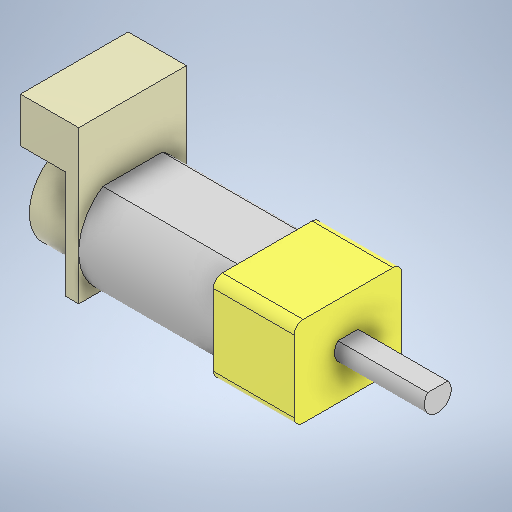
# Autodesk Inventor part: motor
Saved by Autodesk Inventor 2025.2 (Build 292293000, 293)
## iProperties
Created: 2025-06-11
Part Number: motor
Material: Generic
Document SubType Name: Modeling
Designer: cdavi
Density: 1 g/cm^3
Appearance: Default
Author: cdavi
Autodesk Inventor part; units mm, degrees
ref_plane "YZ Plane" through (0, 0, 0) normal (1, 0, 0) x (0, 1, 0)
ref_plane "XZ Plane" through (0, 0, 0) normal (0, 1, 0) x (-1, 0, 0)
ref_plane "XY Plane" through (0, 0, 0) normal (0, 0, 1) x (1, 0, 0)
sketch "Sketch1" plane through (0, 0, 0) normal (0, 1, 0) x (-1, 0, 0)
  line L0 (7.5, 6) -> (-7.5, 6)
  line L1 (-7.5, 6) -> (-7.5, -6)
  line L2 (-7.5, -6) -> (7.5, -6)
  line L3 (7.5, -6) -> (7.5, 6)
  line L4 (7.5, 6) -> (-7.5, -6) construction
  line L5 (-7.5, 6) -> (7.5, -6) construction
  line L6 (7.5, 6) -> (14, 6)
  line L7 (14, 6) -> (14, -6)
  line L8 (14, -6) -> (7.5, -6)
  line L9 (7.5, -6) -> (7.5, 6)
  line L10 (-7.5, 6) -> (-16.5, 6)
  line L11 (-16.5, 6) -> (-16.5, -6)
  line L12 (-16.5, -6) -> (-7.5, -6)
  line L13 (-7.5, -6) -> (-7.5, 6)
  point P0 (0, 0)
  dimension "d0" = 6.5
  dimension "d1" = 12
  dimension "d2" = 9
  dimension "d3" = 21.5
  constraints: 28 end point, 6 parallel, 3 horizontal, 3 perpendicular, 2 collinear, 2 midpoint
  measures "d0" distance between parallel lines of L3 L7
  measures "d1" distance of L6.end L7.end
  measures "d2" distance between parallel lines of L11 L1
  measures "d3" distance between parallel lines of L7 L1
extrude "Extrusion1" add sketch "Sketch1" along normal blind 17 contours L6 L7 L8 L3
extrude "Extrusion2" add sketch "Sketch1" along normal blind 10 separate body contours L3 L2 L1 L0
extrude "Extrusion3" add sketch "Sketch1" along normal blind 10 separate body contours L1 L12 L11 L10
sketch "Sketch2" plane through (16.5, 0, 6) normal (1, 0, 0) x (0, 0, -1)
  circle A0 centre (6, 5) radius 1.5
  line L0 (0, 0) -> (0, 17) projected
  line L1 (4.882, 6) -> (7.118, 6)
  line L2 (12, 10) -> (0, 10) projected
  line L3 (12, 0) -> (0, 0) projected
  line L4 (0, 10) -> (0, 0)
  point P0 (6, 0)
  point P1 (0, 5)
  point P2 (6, 6)
  dimension "d10" = 3
  dimension "d11" = 1
  dimension "d12" = 5
  constraints: 4 end point, 2 point on circle, 1 centre point, 1 horizontal, 1 horizontal alignment, 1 midpoint, 1 point on line, 1 vertical, 1 vertical alignment
  measures "d10" diameter of A0
  measures "d11" distance of point (6, 6) A0.centre
  measures "d12" distance from line of L3 point (0, 5)
extrude "Extrusion4" add sketch "Sketch2" along normal blind 10 separate body contours A0 L1 picked at (6.0594, 5.1702)
sketch "Sketch3" plane through (-14, 0, -6) normal (-1, 0, 0) x (0, 0, 1)
  line L0 (0, 0) -> (0, 17) projected
  line L1 (0, 12) -> (12, 12)
  line L2 (12, 0) -> (12, 17) projected
  line L3 (0, 17) -> (12, 17) projected
  arc A0 (4.882, 6) -> (7.118, 6) centre (6, 5) ccw projected
  circle A1 centre (6, 5) radius 5
  line L4 (0, 12) -> (0, 0)
  line L5 (12, 0) -> (12, 12)
  line L6 (12, 12) -> (12, 0)
  line L7 (0, 0) -> (12, 0)
  line L8 (0, 0) -> (0, 12)
  point P0 (6, 0)
  point P1 (6, 0)
  dimension "d15" = 5
  dimension "d16" = 10
  constraints: 12 end point, 3 collinear, 2 point on line, 1 centre point, 1 coincident, 1 horizontal, 1 perpendicular, 1 vertical
  measures "d15" distance between parallel lines of L1 L3
  measures "d16" diameter of A1
extrude "Extrusion5" cut sketch "Sketch3" against normal blind 5 contours L0 L1 L2 L7 bodies 1
fillet "Fillet1" radius 1 4 edges at (12, 0, 6) (12, 10, 6) (12, 10, -6) (12, 0, -6)
sketch "Sketch4" plane through (7.5, 0, 6) normal (1, 0, 0) x (0, 0, -1)
  arc A0 (4.882, 6) -> (7.118, 6) centre (6, 5) ccw projected
  circle A1 centre (6, 5) radius 6
  line L0 (0, 0) -> (0, 17) projected
  line L1 (0, 10.0481) -> (0, 0)
  line L2 (0, 0) -> (13.8807, 0)
  line L3 (0, 0) -> (12, 0)
  line L4 (12, 0) -> (12, 17) projected
  line L5 (0, 10) -> (12, 10) projected
  line L6 (0, 0) -> (12, 0) projected
  line L7 (12, 0) -> (12, 10) projected
  line L8 (0, 10) -> (12, 10) projected
  line L9 (0, 0) -> (0, 10) projected
  point P0 (6, 0)
  point P1 (2.6834, 10)
  point P2 (0, 5)
  point P3 (2.6834, 0)
  point P4 (9.3166, 10)
  point P5 (12, 5)
  point P6 (9.3166, 0)
  dimension "d20" = 12
  constraints: 6 end point, 2 point on line, 1 centre point, 1 coincident, 1 collinear, 1 perpendicular
  measures "d20" diameter of A1
extrude "Extrusion6" cut sketch "Sketch4" against normal up to next contours L4 L2 A1 | A1 L5 L4 | A1 L0 L5 | L2 L0 A1 bodies 2
equation "\"d12\" = 0.5 * d8"
equation "\"d8\" = 10"
body "Solid1"
body "Solid2"
body "Solid3"
body "Solid4"
